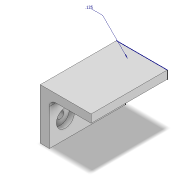
# Autodesk Inventor part: Gyro Mount
Saved by Autodesk Inventor 2020 (Build 240168000, 168)
## iProperties
Created: 2019-08-21
Part Number: Gyro Mount
Material: Generic
Document SubType Name: Modeling
Designer: chitl
Density: 1 g/cm^3
Appearance: Default
Author: chitl
Autodesk Inventor part; units mm, degrees
ref_plane "YZ Plane" through (0, 0, 0) normal (1, 0, 0) x (0, 1, 0)
ref_plane "XZ Plane" through (0, 0, 0) normal (0, 1, 0) x (-1, 0, 0)
ref_plane "XY Plane" through (0, 0, 0) normal (0, 0, 1) x (1, 0, 0)
sketch "Sketch1" plane through (0, 0, 0) normal (0, 0, 1) x (1, 0, 0)
  line L0 (0, 0) -> (25.4, 0)
  line L1 (25.4, 0) -> (25.4, -4.0087)
  line L2 (0, -25.4) -> (0, 0)
  line L3 (4.5437, -25.4) -> (0, -25.4)
  line L4 (4.5437, -25.4) -> (4.5437, -7.1837)
  line L5 (7.7187, -4.0087) -> (25.4, -4.0087)
  arc A0 (7.7187, -4.0087) -> (4.5437, -7.1837) centre (7.7187, -7.1837) ccw
  dimension "d3" = 3.175
  constraints: 12 end point, 2 parallel, 2 perpendicular, 2 point on circle, 2 tangent, 1 centre point, 1 horizontal, 1 vertical
  measures "d3" radius of A0
extrude "Extrusion1" add sketch "Sketch1" along normal blind 38.1
sketch "Sketch2" plane through (4.5437, -25.4, 0) normal (1, 0, 0) x (0, 0, -1)
  circle A0 centre (-30.1153, 9.3268) radius 1.75
  circle A1 centre (-8.7049, 9.5453) radius 1.75
  point P0 (0, 25.4)
  dimension "d6" = 3.5
  dimension "d7" = 3.5
  constraints: 2 centre point, 2 coincident
  measures "d6" diameter of A0
  measures "d7" diameter of A1
extrude "Extrusion2" cut sketch "Sketch2" against normal blind 38.1
hole "Hole1" at (4.5437, -16.0732, 30.1153) at (4.5437, -15.8547, 8.7049) direction (-1, 0, 0) diameter 9 depth 2.54
body "Solid1"
